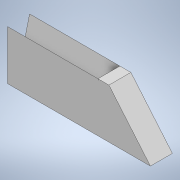
# Autodesk Inventor part: edge holder tip
Saved by Autodesk Inventor 2021 (Build 250183000, 183)
## iProperties
Created: 2021-06-29
Part Number: edge holder tip
Material: Generic
Document SubType Name: Modeling
Designer: newic
Density: 1 g/cm^3
Appearance: Default
Author: newic
Autodesk Inventor part; units mm, degrees
ref_plane "YZ Plane" through (0, 0, 0) normal (1, 0, 0) x (0, 1, 0)
ref_plane "XZ Plane" through (0, 0, 0) normal (0, 1, 0) x (-1, 0, 0)
ref_plane "XY Plane" through (0, 0, 0) normal (0, 0, 1) x (1, 0, 0)
sketch "Sketch1" plane through (0, 0, 0) normal (1, 0, 0) x (0, 1, 0)
  line L0 (0, 0) -> (3.175, 0)
  line L1 (3.175, -12.7) -> (0, -12.7)
  line L2 (0, -12.7) -> (0, 0)
  line L3 (3.175, 0) -> (28.575, 0)
  line L4 (3.175, -12.7) -> (28.575, -12.7)
  line L5 (12.065, -4.1275) -> (28.575, 0)
  line L6 (12.065, -8.5725) -> (28.575, -12.7)
  line L7 (12.065, -4.1275) -> (3.175, -4.1275)
  line L8 (12.065, -8.5725) -> (3.175, -8.5725)
  line L9 (3.175, -4.1275) -> (2.54, -4.1275)
  line L10 (2.54, -4.1275) -> (2.54, -8.5725)
  line L11 (2.54, -8.5725) -> (3.175, -8.5725)
  dimension "d0" = 3.175
  dimension "d1" = 12.7
  dimension "d2" = 25.4
  dimension "d3" = 0.635
  constraints: 24 end point, 3 horizontal, 1 parallel, 1 perpendicular, 1 vertical
  measures "d0" distance of L1.start L1.end
  measures "d1" distance of L0.end L1.start
  measures "d2" distance of L0.end L3.end
  measures "d3" distance of L7.end L9.end
extrude "Extrusion1" add sketch "Sketch1" along normal blind 88.9
sketch "Sketch2" plane through (0, 0, 0) normal (0, 0, 1) x (1, 0, 0)
  line L0 (70.7723, 45.5937) -> (70.7723, 36.3388)
  line L1 (0, 12.065) -> (88.9, 12.065) projected
  line L2 (70.7723, 36.3388) -> (70.7723, 45.5937)
  line L3 (70.7723, 45.5937) -> (88.9, 45.5937)
  line L4 (88.9, 45.5937) -> (70.7723, 45.5937)
  line L5 (70.7723, 45.5937) -> (79.5643, 35.1158)
  line L6 (88.9, 12.065) -> (88.9, 28.575) projected
  line L7 (88.9, 28.575) -> (57.2257, 28.575)
  line L8 (0, 28.575) -> (88.9, 28.575) projected
  line L9 (88.9, 0) -> (76.2, 0)
  line L10 (0, 0) -> (88.9, 0) projected
  line L11 (76.2, 0) -> (52.2227, 28.575)
  line L12 (52.2227, 28.575) -> (52.2227, 24.9497)
  line L13 (0, 28.575) -> (0, 0) projected
  line L14 (0, 0) -> (88.9, 0) projected
  line L15 (88.9, 28.575) -> (88.9, 0) projected
  line L16 (0, 28.575) -> (88.9, 28.575) projected
  dimension "d6" = 40
  dimension "d8" = 12.7
  dimension "d9" = 40
  constraints: 18 end point, 3 point on line, 2 collinear, 1 horizontal, 1 perpendicular, 1 vertical
  measures "d6" angle of L0 L5
  measures "d8" distance of L9.start L9.end
  measures "d9" angle of L11 L12
extrude "Extrusion2" add sketch "Sketch2" against normal blind 12.7 contours L11 L8 L7 L6 L1 | L1 L15 L9 L11
sketch "Sketch3" plane through (0, 0, 0) normal (0, 0, 1) x (1, 0, 0)
  line L0 (0, 28.575) -> (52.2227, 28.575) projected
  line L1 (52.2227, 28.575) -> (58.5727, 28.575)
  line L2 (52.2227, 28.575) -> (88.9, 28.575) projected
  line L3 (52.2227, 28.575) -> (66.0763, 12.065) projected
  line L4 (58.5727, 28.575) -> (89.629, -8.4365)
  line L5 (58.5727, 28.575) -> (106.8878, 28.575) construction
  line L6 (89.629, -8.4365) -> (99.364, 12.7806)
  line L7 (99.364, 12.7806) -> (87.0878, 39.7231)
  line L8 (87.0878, 39.7231) -> (61.7749, 33.0961)
  line L9 (61.7749, 33.0961) -> (58.5727, 28.575)
  point P0 (0, 0)
  dimension "d12" = 6.35
  dimension "d13" = 50
  constraints: 14 end point, 1 equal length, 1 horizontal, 1 point on line
  measures "d12" distance of L0.end L1.end
  measures "d13" angle of L4 L5
extrude "Extrusion3" cut sketch "Sketch3" against normal blind 12.7
body "Solid1"
